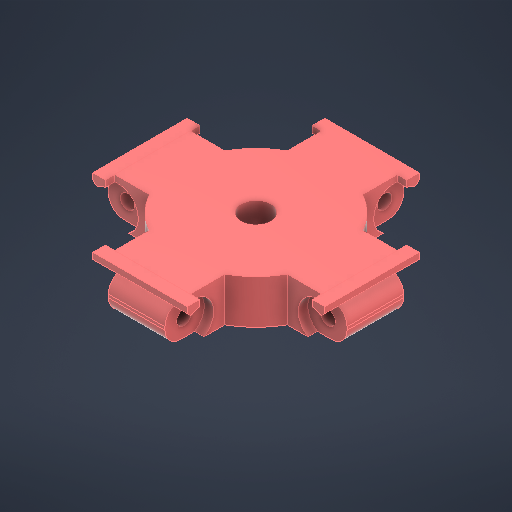
# Autodesk Inventor part: SujeccionHelices
Saved by Autodesk Inventor 2026.1 (Build 301233000, 233)
## iProperties
Created: 2025-11-10
Part Number: SujeccionHelices
Material: PLA
Document SubType Name: Modeling
Designer: vickh
Density: 1.3 g/cm^3
Appearance: Suave - Rojo
Mass: 57.6997 g
Surface Area: 138.679 cm^2
Volume: 44.3844 cm^3
Author: vickh
## iProperties of the stored document SujeccionHelices_3DPrint.ipt
Created: 2025-11-17
Part Number: SujeccionHelices_3DPrint
Material: Genérico
Document SubType Name: Modeling
Designer: usuario
Density: 1 g/cm^3
Appearance: Valor por defecto
Author: usuario
Autodesk Inventor part; units mm, degrees
ref_plane "YZ Plane" through (0, 0, 0) normal (1, 0, 0) x (0, 1, 0)
ref_plane "XZ Plane" through (0, 0, 0) normal (0, 1, 0) x (-1, 0, 0)
ref_plane "XY Plane" through (0, 0, 0) normal (0, 0, 1) x (1, 0, 0)
sketch "Boceto3" plane through (0, 0, 0) normal (0, 1, 0) x (-1, 0, 0)
  line L0 (-50, 50) -> (50, 50) construction
  line L1 (50, 50) -> (50, -50) construction
  line L2 (50, -50) -> (-50, -50) construction
  line L3 (-50, -50) -> (-50, 50) construction
  line L4 (-50, 50) -> (50, -50) construction
  line L5 (50, 50) -> (-50, -50) construction
  circle A0 centre (0, 0) radius 10.25
  dimension "d5" = 100
  dimension "d6" = 100
  dimension "d7" = 20.5
  constraints: 12 end point, 2 midpoint, 2 parallel, 1 centre point, 1 coincident, 1 horizontal, 1 perpendicular
  measures "d5" distance of L1.end L2.end
  measures "d6" distance of L0.end L1.end
  measures "d7" diameter of A0
extrude "Extrusión2" add sketch "Boceto3" along normal blind 10
sketch "Boceto4" plane through (0, 10, 0) normal (0, 1, 0) x (1, 0, 0)
  line L0 (-38, -12) -> (-21.9317, -12)
  line L1 (-21.9317, 12) -> (-38, 12)
  line L2 (-38, 12) -> (-38, -12)
  line L3 (-38, -12) -> (-21.9317, 12) construction
  line L4 (-21.9317, -12) -> (-38, 12) construction
  line L5 (-84.3268, 0) -> (47.4613, 0) construction
  line L6 (-12, -21.9317) -> (-12, -38)
  line L7 (-12, -38) -> (12, -38)
  line L8 (12, -38) -> (12, -21.9317)
  line L9 (21.9317, -12) -> (38, -12)
  line L10 (38, -12) -> (38, 12)
  line L11 (38, 12) -> (21.9317, 12)
  line L12 (12, 21.9317) -> (12, 38)
  line L13 (12, 38) -> (-12, 38)
  line L14 (-12, 38) -> (-12, 21.9317)
  arc A0 (21.9317, 12) -> (12, 21.9317) centre (0, 0) ccw
  arc A1 (-12, 21.9317) -> (-21.9317, 12) centre (0, 0) ccw
  arc A2 (-21.9317, -12) -> (-12, -21.9317) centre (0, 0) ccw
  arc A3 (12, -21.9317) -> (21.9317, -12) centre (0, 0) ccw
  point P0 (-29.9659, 0)
  point P1 (-29.9659, 0)
  point P2 (-38, 0)
  point P3 (-29.9659, -12)
  point P4 (0, -38)
  point P5 (12, -29.9659)
  point P6 (38, 0)
  point P7 (29.9659, 12)
  point P8 (0, 38)
  point P9 (-12, 29.9659)
  dimension "d15" = 38
  dimension "d16" = 24
  dimension "d19" = 360
  dimension "d21" = 25
  constraints: 30 end point, 8 point on circle, 5 midpoint, 4 centre point, 2 horizontal, 2 point on line, 1 coincident, 1 parallel, 1 vertical, 37 other
  measures "d15" distance of point (0, 0) point (-38, 0)
  measures "d16" distance from line of point (-29.966, -12) L1
  measures "d21" radius of A0
extrude "Extrusión3" add sketch "Boceto4" along normal blind 11
sketch "Boceto7" plane through (0, 0, 0) normal (0, -1, 0) x (1, 0, 0)
  circle A0 centre (0, 0) radius 8.15
  dimension "d26" = 16.3
  constraints: 1 centre point, 1 coincident
  measures "d26" diameter of A0
extrude "Extrusión4" cut sketch "Boceto7" against normal blind 5
fillet "Empalme1" radius 5 8 edges at (0, 10, -38) (0, 21, -38) (38, 10, 0) (38, 21, 0) (0, 10, 38) (0, 21, 38) (-38, 10, 0) (-38, 21, 0)
sketch "Boceto9" plane through (-12, 10, 21.9317) normal (-1, 0, 0) x (0, 0, 1)
  line L0 (0, 0) -> (-9.9317, 0) projected
  line L1 (0, 0) -> (16.0683, 0) construction
  line L2 (16.0683, 0) -> (16.0683, 11) construction
  line L3 (16.0683, 11) -> (0, 11) construction
  line L4 (0, 11) -> (0, 0) construction
  line L5 (0, 11) -> (11.0683, 11) construction
  line L6 (16.0683, 11) -> (0, 0) construction
  line L7 (0, 11) -> (16.0683, 0) construction
  line L8 (0, 0) -> (0, 11) construction
  circle A0 centre (10.0341, 5.5) radius 2.25
  line L9 (8.0341, 5.5) -> (16.0683, 5.5) construction
  arc A1 (11.0683, 0) -> (16.0683, 5) centre (11.0683, 5) ccw projected
  point P0 (-21.9317, -10)
  dimension "d31" = 4.5
  dimension "d120" = 2
  constraints: 14 end point, 3 midpoint, 2 parallel, 1 centre point, 1 collinear, 1 horizontal, 1 perpendicular, 1 point on line, 1 tangent
  measures "d31" diameter of A0
  measures "d120" distance of A0.centre point (8.034, 5.5)
sketch "Boceto13" plane through (0, 21, 0) normal (0, 1, 0) x (1, 0, 0)
  line L0 (-33.5, -33.5) -> (33.5, -33.5)
  line L1 (33.5, -33.5) -> (33.5, 33.5)
  line L2 (33.5, 33.5) -> (-33.5, 33.5)
  line L3 (-33.5, 33.5) -> (-33.5, -33.5)
  line L4 (-33.5, -33.5) -> (33.5, 33.5) construction
  line L5 (33.5, -33.5) -> (-33.5, 33.5) construction
  point P0 (0, 0)
  point P1 (0, 0)
  dimension "d118" = 33.5
  dimension "d119" = 33.5
  constraints: 12 end point, 2 midpoint, 2 parallel, 1 horizontal, 1 perpendicular
  measures "d118" distance from line of point (0, 0) L2
  measures "d119" distance from line of L1 point (0, 0)
sweep "Barrido1" cut profiles "Boceto9" path "Boceto13" path curves L3 L0 L1 L2
sketch "Boceto19" plane through (0, 21, 0) normal (0, 1, 0) x (1, 0, 0)
  circle A0 centre (0, 0) radius 4.75
  dimension "d63" = 9.5
  constraints: 1 centre point, 1 coincident
  measures "d63" diameter of A0
extrude "Extrusión13" cut sketch "Boceto19" against normal blind 10
sketch "Boceto22" plane through (0, 21, 0) normal (0, 1, 0) x (1, 0, 0)
  line L0 (21.9317, -12) -> (33, -12) projected
  line L1 (38, -12) -> (38, 12) projected
  line L2 (36.9317, 15) -> (21.9317, 15)
  line L3 (21.9317, 15) -> (21.9317, -15)
  line L4 (21.9317, -15) -> (36.9317, -15)
  line L5 (36.9317, -15) -> (36.9317, 15)
  line L6 (21.9317, 12) -> (21.9317, -12) construction
  line L7 (21.9317, 12) -> (21.9317, -12) construction
  line L8 (21.9317, -12) -> (38, -12) construction
  line L9 (38, -12) -> (38, 12) construction
  line L10 (38, 12) -> (21.9317, 12) construction
  line L11 (21.9317, 12) -> (38, -12) construction
  line L12 (21.9317, -12) -> (38, 12) construction
  line L13 (35.9659, 15) -> (32.9659, 15)
  line L14 (32.9659, 15) -> (32.9659, -15)
  line L15 (32.9659, -15) -> (35.9659, -15)
  line L16 (35.9659, -15) -> (35.9659, 15)
  circle A0 centre (0, 0) radius 4.75 projected
  line L17 (15, 32.9659) -> (15, 35.9659)
  line L18 (15, 21.9317) -> (15, 36.9317)
  line L19 (12, 21.9317) -> (12, 38)
  line L20 (-15, 21.9317) -> (15, 21.9317)
  line L21 (12, 21.9317) -> (-12, 38) construction
  line L22 (-12, 21.9317) -> (12, 21.9317) construction
  line L23 (-12, 21.9317) -> (12, 21.9317) construction
  line L24 (12, 38) -> (-12, 38)
  line L25 (-12, 21.9317) -> (12, 38) construction
  line L26 (15, 35.9659) -> (-15, 35.9659)
  line L27 (-15, 32.9659) -> (15, 32.9659)
  line L28 (15, 36.9317) -> (-15, 36.9317)
  line L29 (-12, 38) -> (-12, 21.9317)
  line L30 (-15, 35.9659) -> (-15, 32.9659)
  line L31 (-15, 36.9317) -> (-15, 21.9317)
  line L32 (-32.9659, 15) -> (-35.9659, 15)
  line L33 (-21.9317, 15) -> (-36.9317, 15)
  line L34 (-21.9317, 12) -> (-38, 12) construction
  line L35 (-21.9317, -15) -> (-21.9317, 15)
  line L36 (-21.9317, 12) -> (-38, -12) construction
  line L37 (-21.9317, -12) -> (-21.9317, 12) construction
  line L38 (-21.9317, -12) -> (-21.9317, 12) construction
  line L39 (-38, 12) -> (-38, -12) construction
  line L40 (-21.9317, -12) -> (-38, 12) construction
  line L41 (-35.9659, 15) -> (-35.9659, -15)
  line L42 (-32.9659, -15) -> (-32.9659, 15)
  line L43 (-36.9317, 15) -> (-36.9317, -15)
  line L44 (-38, -12) -> (-21.9317, -12) construction
  line L45 (-35.9659, -15) -> (-32.9659, -15)
  line L46 (-36.9317, -15) -> (-21.9317, -15)
  line L47 (-15, -32.9659) -> (-15, -35.9659)
  line L48 (-15, -21.9317) -> (-15, -36.9317)
  line L49 (-12, -21.9317) -> (-12, -38)
  line L50 (15, -21.9317) -> (-15, -21.9317)
  line L51 (-12, -21.9317) -> (12, -38) construction
  line L52 (12, -21.9317) -> (-12, -21.9317) construction
  line L53 (12, -21.9317) -> (-12, -21.9317) construction
  line L54 (-12, -38) -> (12, -38)
  line L55 (12, -21.9317) -> (-12, -38) construction
  line L56 (-15, -35.9659) -> (15, -35.9659)
  line L57 (15, -32.9659) -> (-15, -32.9659)
  line L58 (-15, -36.9317) -> (15, -36.9317)
  line L59 (12, -38) -> (12, -21.9317)
  line L60 (15, -35.9659) -> (15, -32.9659)
  line L61 (15, -36.9317) -> (15, -21.9317)
  line L62 (12, -33) -> (12, -21.9317) projected
  line L63 (-12, -21.9317) -> (-12, -33) projected
  line L64 (-33, -12) -> (-21.9317, -12) projected
  circle A1 centre (0, 0) radius 4.75 projected
  line L65 (12, -33) -> (12, -21.9317) projected
  arc A2 (12, -21.9317) -> (21.9317, -12) centre (0, 0) ccw projected
  line L66 (21.9317, -12) -> (33, -12) projected
  line L67 (33, 12) -> (33, -12) projected
  line L68 (33, 12) -> (21.9317, 12) projected
  arc A3 (21.9317, 12) -> (12, 21.9317) centre (0, 0) ccw projected
  line L69 (12, 21.9317) -> (12, 33) projected
  line L70 (-12, 33) -> (12, 33) projected
  line L71 (-12, 33) -> (-12, 21.9317) projected
  arc A4 (-12, 21.9317) -> (-21.9317, 12) centre (0, 0) ccw projected
  line L72 (-21.9317, 12) -> (-33, 12) projected
  line L73 (-33, -12) -> (-33, 12) projected
  line L74 (-33, -12) -> (-21.9317, -12) projected
  arc A5 (-21.9317, -12) -> (-12, -21.9317) centre (0, 0) ccw projected
  line L75 (-12, -21.9317) -> (-12, -33) projected
  line L76 (12, -33) -> (-12, -33) projected
  point P0 (47.7963, -3.2782)
  point P1 (33.5, 12)
  point P2 (29.4317, -15)
  point P3 (29.9659, 0)
  point P4 (29.9659, 0)
  point P5 (32.9659, 0)
  point P6 (29.9659, 0)
  point P7 (43.9977, -12)
  point P8 (32.9659, 15)
  point P9 (21.9317, -12)
  point P10 (32.9659, -12)
  point P11 (15, 29.4317)
  point P12 (3.2782, 47.7963)
  point P13 (0, 29.9659)
  point P14 (0, 29.9659)
  point P15 (0, 32.9659)
  point P16 (0, 29.9659)
  point P17 (-12, 38)
  point P18 (-12, 33.5)
  point P19 (-29.4317, 15)
  point P20 (-47.7963, 3.2782)
  point P21 (-29.9659, 0)
  point P22 (-29.9659, 0)
  point P23 (-32.9659, 0)
  point P24 (-29.9659, 0)
  point P25 (-38, -12)
  point P26 (-33.5, -12)
  point P27 (-15, -29.4317)
  point P28 (-3.2782, -47.7963)
  point P29 (0, -29.9659)
  point P30 (0, -29.9659)
  point P31 (0, -32.9659)
  point P32 (0, -29.9659)
  point P33 (12, -38)
  point P34 (12, -33.5)
  point P35 (12, 32.9659)
  point P36 (-12, 32.9659)
  point P37 (-12, 21.9317)
  point P38 (12, 21.9317)
  point P39 (-43.9977, -12)
  point P40 (-32.0839, -12)
  point P41 (-35.9659, 15)
  point P42 (-32.9659, -12)
  point P43 (-21.9317, -12)
  point P44 (12, -32.9659)
  point P45 (12, -21.9317)
  point P46 (-12, -21.9317)
  point P47 (-12, -32.9659)
  point P48 (-15, -35.9659)
  point P49 (12, 21.9317)
  point P50 (-15, 32.9659)
  point P51 (-15, -35.9659)
  point P52 (15, -32.9659)
  point P53 (12, 32.9659)
  point P54 (-12, 32.9659)
  point P55 (-12, -32.9659)
  point P56 (12, -32.9659)
  point P57 (-12, -32.9659)
  point P58 (-32.9659, 12)
  point P59 (12, -32.9659)
  point P60 (32.9659, 12)
  dimension "d75" = 30
  dimension "d76" = 15
  dimension "d77" = 15
  dimension "d83" = 3
  dimension "d84" = 3
  dimension "d91" = 360
  dimension "d117" = 12
  constraints: 120 end point, 12 midpoint, 8 point on line, 6 parallel, 4 collinear, 3 horizontal, 3 perpendicular, 1 vertical, 155 other
  measures "d75" distance of L4.end L2.start
  measures "d76" distance between parallel lines of L3 L5
  measures "d77" vertical distance of point (29.432, -15) point (29.966, 0)
  measures "d83" distance of L15.end L14.end
  measures "d84" distance of point (32.966, 0) point (29.966, 0)
sketch "Boceto18" plane through (12, 10, 21.9317) normal (1, 0, 0) x (0, 0, -1)
  circle A0 centre (-10.0341, 5.5) radius 2.25 projected
  circle A1 centre (53.8976, 5.5) radius 2.25 projected
  circle A2 centre (-10.0341, 5.5) radius 6.5
  circle A3 centre (53.8976, 5.5) radius 6.5
  point P0 (21.9317, -10)
  dimension "d59" = 13
  dimension "d60" = 13
  constraints: 2 centre point, 2 coincident
  measures "d59" diameter of A2
  measures "d60" diameter of A3
sketch "Boceto15" plane through (-21.9317, 10, 12) normal (0, 0, 1) x (1, 0, 0)
  circle A0 centre (-10.0341, 5.5) radius 2.25 projected
  circle A1 centre (-10.0341, 5.5) radius 6.5
  circle A2 centre (53.8976, 5.5) radius 2.25 projected
  circle A3 centre (53.8976, 5.5) radius 6.5
  point P0 (21.9317, -10)
  dimension "d47" = 13
  dimension "d54" = 13
  constraints: 2 centre point, 2 coincident
  measures "d47" diameter of A1
  measures "d54" diameter of A3
sketch "Boceto17" plane through (-12, 10, 21.9317) normal (-1, 0, 0) x (0, 0, 1)
  circle A0 centre (10.0341, 5.5) radius 2.25 projected
  circle A1 centre (-53.8976, 5.5) radius 2.25 projected
  circle A2 centre (-53.8976, 5.5) radius 6.5
  circle A3 centre (10.0341, 5.5) radius 6.5
  point P0 (-21.9317, -10)
  dimension "d55" = 13
  dimension "d56" = 13
  constraints: 2 centre point, 2 coincident
  measures "d55" diameter of A2
  measures "d56" diameter of A3
extrude "Extrusión21" add sketch "Boceto22" along normal blind 3 contours L3 L68 L14 L0 | A2 L50 A5 L35 A4 L20 A3 L3 | L0 L67 L68 L14 L2 L16 L4 | L59 L57 L49 L50 | L20 L29 L27 L19 | L57 L60 L56 L59 | L16 L2 L5 L4 | L27 L29 L70 L19 | L19 L26 L17 L27 | L49 L56 L47 L57 | L64 L42 L72 L35 | L59 L56 L49 L76 | L70 L29 L26 L19 | L27 L30 L26 L29 | L61 L58 L59 L56 | L42 L45 L41 L32 L72 L73 L64 | L59 L58 L49 L56 | L26 L29 L28 L19 | L19 L28 L18 L26 | L49 L58 L48 L56 | L26 L31 L28 L29 | L46 L43 L33 L41
extrude "Extrusión18" cut sketch "Boceto17" along normal mid plane 6
extrude "Extrusión19" cut sketch "Boceto15" along normal mid plane 6
extrude "Extrusión20" cut sketch "Boceto18" along normal mid plane 6
sketch "Boceto23" plane through (21.9317, 10, -12) normal (0, 0, -1) x (-1, 0, 0)
  circle A0 centre (-10.0341, 5.5) radius 6.5
  circle A1 centre (53.8976, 5.5) radius 6.5
  point P0 (21.9317, -10)
  point P1 (-10.0341, 5.5)
  point P2 (53.8976, 5.5)
  dimension "d94" = 13
  dimension "d95" = 13
  constraints: 2 centre point, 2 coincident
  measures "d94" diameter of A0
  measures "d95" diameter of A1
extrude "Extrusión17" cut sketch "Boceto23" along normal mid plane 6
sketch "Boceto25" plane through (0, 24, 0) normal (0, 1, 0) x (1, 0, 0)
  circle A0 centre (0, 0) radius 8.15 projected
  circle A1 centre (0, 0) radius 45
  dimension "d110" = 90
  constraints: 1 centre point, 1 coincident
  measures "d110" diameter of A1
chamfer "Chaflán1" distance 1 angle 45 4 edges at (0, 21, 36.9317) (36.9317, 21, 0) (0, 21, -36.9317) (-36.9317, 21, 0)
chamfer "Chaflán2" distance 3 angle 45 1 edges at (10.25, 10, 0)
